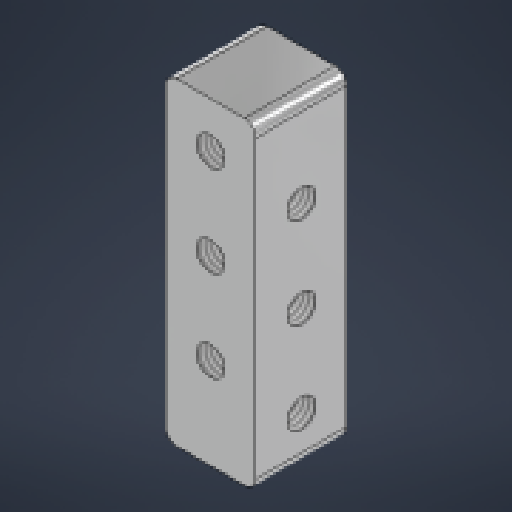
# Autodesk Inventor part: PLATE,NUT-BLOCK,3-LONG
Saved by Autodesk Inventor 2026.1 (Build 301233020, 233B)
## iProperties
Created: 2026-02-08
Part Number: PLATE,NUT-BLOCK,3-LONG
Material: Aluminum 6061
Document SubType Name: Sheet Metal
Designer: Owen L
Density: 2.7 g/cm^3
Sheet Metal Rule: Default
Appearance: Aluminum - Flat
Author: Owen L
Autodesk Inventor part; units mm, degrees
ref_plane "YZ Plane" through (0, 0, 0) normal (1, 0, 0) x (0, 1, 0)
ref_plane "XZ Plane" through (0, 0, 0) normal (0, 1, 0) x (-1, 0, 0)
ref_plane "XY Plane" through (0, 0, 0) normal (0, 0, 1) x (1, 0, 0)
sketch "Sketch1" plane through (0, 0, 0) normal (0, 0, 1) x (1, 0, 0)
  line L0 (6.35, -22.225) -> (-6.35, -22.225)
  line L1 (-6.35, -22.225) -> (-6.35, 22.225)
  line L2 (-6.35, 22.225) -> (6.35, 22.225)
  line L3 (6.35, 22.225) -> (6.35, -22.225)
  line L4 (6.35, -22.225) -> (-6.35, 22.225) construction
  line L5 (-6.35, -22.225) -> (6.35, 22.225) construction
  point P0 (0, 0)
  dimension "d0" = 12.7
  dimension "d6" = 44.45
  measures "d0" distance of L1.end L2.end
  measures "d6" distance of L0.end L1.end
extrude "Plate1" add sketch "Sketch1" along normal blind 12.7
sketch "Sketch2" plane through (6.35, -22.225, 0) normal (1, 0, 0) x (0, 0, -1)
  line L0 (0, 0) -> (-12.7, 0) projected
  line L1 (0, 0) -> (0, 44.45) projected
  point P0 (0, 22.225)
  point P1 (-6.35, 6.35)
  point P2 (-6.35, 19.05)
  point P3 (-6.35, 31.75)
  dimension "d2" = 6.35
  dimension "d3" = 12.7
  dimension "d4" = 12.7
  dimension "d5" = 6.35
  constraints: 2 vertical alignment
  measures "d2" distance from line of L0 point (-6.35, 6.35)
  measures "d3" distance of point (-6.35, 19.05) point (-6.35, 6.35)
  measures "d4" distance of point (-6.35, 31.75) point (-6.35, 19.05)
  measures "d5" distance from line of L1 point (-6.35, 6.35)
hole "Hole1" at (6.35, -15.875, 6.35) at (6.35, -3.175, 6.35) at (6.35, 9.525, 6.35) direction (-1, 0, 0) diameter 3.9624 depth 12.7 tip angle 118 thread size "10-32 UNF" class "2B" standard "ANSI Unified Screw Threads"
sketch "Sketch3" plane through (0, 0, 12.7) normal (0, 0, 1) x (1, 0, 0)
  line L0 (-6.35, 22.225) -> (6.35, 22.225) projected
  point P0 (0, 0)
  point P1 (0, -9.525)
  point P2 (0, 3.175)
  point P3 (0, 15.875)
  dimension "d14" = 12.7
  dimension "d15" = 12.7
  dimension "d16" = 6.35
  constraints: 3 vertical alignment
  measures "d14" distance of point (0, 3.175) point (0, -9.525)
  measures "d15" distance of point (0, 15.875) point (0, 3.175)
  measures "d16" distance from line of L0 point (0, 15.875)
hole "Hole2" at (0, -9.525, 12.7) at (0, 3.175, 12.7) at (0, 15.875, 12.7) direction (0, 0, -1) diameter 3.9624 depth 12.7 tip angle 118 thread size "10-32 UNF" class "2B" standard "ANSI Unified Screw Threads"
fillet "Corner Round1" radius 1.5875 4 edges at (6.35, -22.225, 6.35) (-6.35, -22.225, 6.35) (6.35, 22.225, 6.35) (-6.35, 22.225, 6.35)
equation "\"d22\" = Thickness"
equation "\"d1\" = Thickness"
equation "\"BendRadius\" = Thickness"
equation "\"BendReliefWidth\" = Thickness"
equation "\"BendReliefDepth\" = 0.5 * Thickness"
equation "\"CornerReliefSize\" = 4 * Thickness"
equation "\"MinimumRemnant\" = 2 * Thickness"
equation "\"TransitionRadius\" = BendRadius"
equation "\"JacobiRadiusSize\" = BendRadius"
equation "\"GapSize\" = Thickness"
equation "\"Thickness\" = 12.7"
body "Solid1"
